Autodesk Inventor part; units mm, degrees
(part 2 of 2)
sketch "Sketch63" plane through (-55, 164.1154, 85) normal (0, 0, 1) x (1, 0, 0)
  circle A0 centre (-4.4646, 400) radius 1.5 projected
  line L0 (31.8727, 516.2941) -> (-4.8296, 379.3193) projected
  arc A1 (36.7023, 520) -> (31.8727, 516.2941) centre (36.7023, 515) ccw projected
  line L1 (73.2977, 520) -> (36.7023, 520) projected
  arc A2 (78.1273, 516.2941) -> (73.2977, 520) centre (73.2977, 515) ccw projected
  line L2 (114.8296, 379.3193) -> (78.1273, 516.2941) projected
  arc A3 (115, 378.0252) -> (114.8296, 379.3193) centre (110, 378.0252) ccw projected
  line L3 (115, 15) -> (115, 378.0252) projected
  arc A4 (110, 10) -> (115, 15) centre (110, 15) ccw projected
  line L4 (0, 10) -> (110, 10) projected
  arc A5 (-5, 15) -> (0, 10) centre (0, 15) ccw projected
  line L5 (-5, 378.0252) -> (-5, 15) projected
  arc A6 (-4.8296, 379.3193) -> (-5, 378.0252) centre (0, 378.0252) ccw projected
  line L6 (22.2134, 518.8823) -> (-14.4889, 381.9075) projected
  arc A7 (-14.4889, 381.9075) -> (-15, 378.0252) centre (0, 378.0252) ccw projected
  line L7 (-15, 378.0252) -> (-15, 15) projected
  arc A8 (-15, 15) -> (0, 0) centre (0, 15) ccw projected
  line L8 (0, 0) -> (110, 0) projected
  arc A9 (110, 0) -> (125, 15) centre (110, 15) ccw projected
  line L9 (125, 15) -> (125, 378.0252) projected
  arc A10 (125, 378.0252) -> (124.4889, 381.9075) centre (110, 378.0252) ccw projected
  line L10 (124.4889, 381.9075) -> (87.7866, 518.8823) projected
  arc A11 (87.7866, 518.8823) -> (73.2977, 530) centre (73.2977, 515) ccw projected
  line L11 (73.2977, 530) -> (36.7023, 530) projected
  arc A12 (36.7023, 530) -> (22.2134, 518.8823) centre (36.7023, 515) ccw projected
  circle A13 centre (104.1119, 438.637) radius 1.5 projected
  circle A14 centre (93.7591, 477.2741) radius 1.5 projected
  circle A15 centre (83.4063, 515.9111) radius 1.5 projected
  circle A16 centre (114.4646, 400) radius 1.5 projected
  circle A17 centre (5, 5) radius 1.5 projected
  circle A18 centre (75, 5) radius 1.5 projected
  circle A19 centre (-10, 300) radius 1.5 projected
  circle A20 centre (-10, 260) radius 1.5 projected
  circle A21 centre (-10, 220) radius 1.5 projected
  circle A22 centre (-10, 180) radius 1.5 projected
  circle A23 centre (-10, 140) radius 1.5 projected
  circle A24 centre (-10, 100) radius 1.5 projected
  circle A25 centre (120, 100) radius 1.5 projected
  circle A26 centre (-10, 60) radius 1.5 projected
  circle A27 centre (120, 60) radius 1.5 projected
  circle A28 centre (-10, 20) radius 1.5 projected
  circle A29 centre (120, 20) radius 1.5 projected
  circle A30 centre (120, 140) radius 1.5 projected
  circle A31 centre (120, 180) radius 1.5 projected
  circle A32 centre (120, 220) radius 1.5 projected
  circle A33 centre (120, 260) radius 1.5 projected
  circle A34 centre (120, 300) radius 1.5 projected
  circle A35 centre (105, 5) radius 1.5 projected
  circle A36 centre (35, 5) radius 1.5 projected
  circle A37 centre (120, 380) radius 1.5 projected
  circle A38 centre (-10, 340) radius 1.5 projected
  circle A39 centre (120, 340) radius 1.5 projected
  circle A40 centre (-10, 380) radius 1.5 projected
  circle A41 centre (5.8881, 438.637) radius 1.5 projected
  circle A42 centre (16.2409, 477.2741) radius 1.5 projected
  circle A43 centre (26.5937, 515.9111) radius 1.5 projected
  circle A44 centre (55, 525) radius 1.5 projected
  point P0 (55, -164.1154)
  constraints: 1 coincident
hole "Hole30" at (-20, 169.1154, 85) at (20, 169.1154, 85) at (50, 169.1154, 85) at (65, 184.1154, 85) at (-50, 169.1154, 85) at (-65, 184.1154, 85) at (-65, 224.1154, 85) at (65, 224.1154, 85) at (65, 264.1154, 85) at (65, 304.1154, 85) at (65, 344.1154, 85) at (65, 384.1154, 85) at (65, 424.1154, 85) at (65, 464.1154, 85) at (65, 504.1154, 85) at (65, 544.1154, 85) at (59.4646, 564.1154, 85) at (49.1119, 602.7525, 85) at (38.7591, 641.3895, 85) at (28.4063, 680.0265, 85) at (0, 689.1154, 85) at (-28.4063, 680.0265, 85) at (-38.7591, 641.3895, 85) at (-49.1119, 602.7525, 85) at (-59.4646, 564.1154, 85) at (-65, 544.1154, 85) at (-65, 504.1154, 85) at (-65, 464.1154, 85) at (-65, 424.1154, 85) at (-65, 384.1154, 85) at (-65, 344.1154, 85) at (-65, 304.1154, 85) at (-65, 264.1154, 85) direction (0, 0, -1) diameter 3.242 depth 11.8 tip angle 118 bodies 9
body "Solid3"
body "Solid12"
body "Solid25"
body "Solid26"
body "Solid27"
body "Solid29"
body "Solid18"
body "Solid19"
body "Solid20"
body "Solid23"
